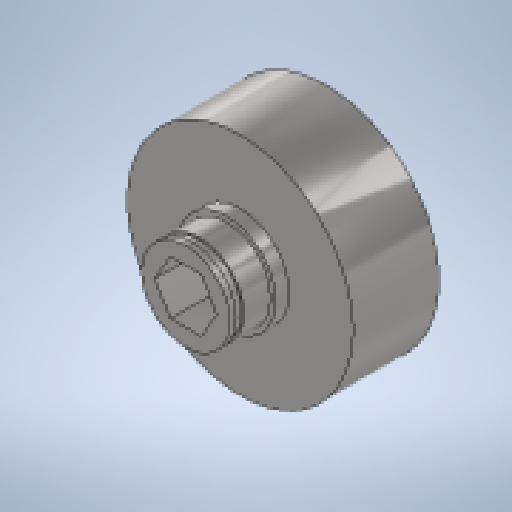
# Autodesk Inventor part: Clutch
Saved by Autodesk Inventor 2023.2 (Build 272271000, 271)
## iProperties
Created: 2024-03-17
Part Number: Clutch
Material: Stainless Steel
Document SubType Name: Modeling
Designer: Nathan Cai
Mass: 40.0707 g
Surface Area: 43.4565 cm^2
Volume: 5.00884 cm^3
Density: 8 g/cm^3
Appearance: Semi-Polished
Author: Nathan Cai
Autodesk Inventor part; units mm, degrees
ref_plane "YZ Plane" through (0, 0, 0) normal (1, 0, 0) x (0, 1, 0)
ref_plane "XZ Plane" through (0, 0, 0) normal (0, 1, 0) x (-1, 0, 0)
ref_plane "XY Plane" through (0, 0, 0) normal (0, 0, 1) x (1, 0, 0)
sketch "Sketch1" plane through (0, 0, 0) normal (1, 0, 0) x (0, 1, 0)
  line L0 (0, 0) -> (15.875, 0) construction
  line L1 (15.875, 0) -> (15.875, 9.525) construction
  line L2 (15.875, 9.525) -> (0, 9.525)
  line L3 (0, 9.525) -> (0, 0) construction
  line L4 (15.875, 0) -> (13.7634, 9.525)
  line L5 (0, 0) -> (16.6688, 0)
  line L6 (16.6688, 0) -> (16.6687, 12.7)
  line L7 (16.6687, 12.7) -> (0, 12.7)
  line L8 (0, 12.7) -> (0, 0)
  line L9 (0, 9.525) -> (6.5, 9.525)
  line L10 (6.5, 9.525) -> (6.5, 20.7266)
  line L11 (6.5, 20.7266) -> (0, 20.7266)
  line L12 (0, 20.7266) -> (0, 9.525)
  line L13 (0, 0) -> (3.9688, 0)
  line L14 (3.9688, 0) -> (3.9687, 20.7266)
  line L15 (3.9687, 20.7266) -> (0, 20.7266)
  line L16 (0, 20.7266) -> (0, 0)
  line L17 (6.5, 19.8) -> (6.2, 19.8)
  line L18 (6.2, 19.8) -> (6.2, 18.7)
  line L19 (6.2, 18.7) -> (6.5, 18.7)
  line L20 (6.5, 18.7) -> (6.5, 19.8)
  line L21 (6.5, 12.7) -> (7.25, 12.7)
  line L22 (7.25, 12.7) -> (7.25, 14.7)
  line L23 (7.25, 14.7) -> (6.5, 14.7)
  line L24 (6.5, 14.7) -> (6.5, 12.7)
  point P0 (3.9687, 9.525)
  dimension "d0" = 15.875
  dimension "d1" = 9.525
  dimension "d2" = 12.5
  dimension "d3" = 0.7937
  dimension "d4" = 12.7
  dimension "d5" = 6.5
  dimension "d6" = 3.9688
  dimension "d7" = 8.0266
  dimension "d8" = 0.3
  dimension "d9" = 1.1
  dimension "d10" = 6
  dimension "d12" = 0.75
  dimension "d13" = 2
  constraints: 50 end point, 12 parallel, 6 horizontal, 6 perpendicular, 5 point on line
  measures "d0" distance of L2.end L1.end
  measures "d1" distance of L1.end L0.end
  measures "d2" angle of L4 L1
  measures "d3" distance between parallel lines of L6 L1
  measures "d4" distance between parallel lines of L0 L7
  measures "d5" distance of L11.end L10.end
  measures "d6" distance between parallel lines of L16 L14
  measures "d7" distance between parallel lines of L7 L11
  measures "d8" distance of L19.end L18.end
  measures "d9" distance of L18.end L17.end
  measures "d10" distance between parallel lines of L7 L19
  measures "d12" distance of L23.end L22.end
  measures "d13" distance of L22.end L21.end
revolve "Revolution1" add sketch "Sketch1" angle 360 about axis through (0, 0, 12.7) along (0, 0, -1) contours L2 L10 L7 L6 L5 L4 | L2 L14 L7 L10 | L10 L23 L22 L7 | L7 L14 L11 L10 L17 L18 L19
sketch "Sketch2" plane through (0, 0, 20.7266) normal (0, 0, 1) x (1, 0, 0)
  circle A0 centre (0, 0) radius 3.9688 construction
  line L0 (2.2914, 3.9688) -> (4.5827, 0)
  line L1 (4.5827, 0) -> (2.2914, -3.9688)
  line L2 (2.2914, -3.9688) -> (-2.2914, -3.9687)
  line L3 (-2.2914, -3.9687) -> (-4.5827, 0)
  line L4 (-4.5827, 0) -> (-2.2914, 3.9688)
  line L5 (-2.2914, 3.9688) -> (2.2914, 3.9688)
  point P0 (0, 0)
  point P1 (0, 0)
  point P2 (0, 3.9687)
  constraints: 12 end point, 1 coincident, 1 horizontal, 1 midpoint, 1 vertical alignment, 14 other
extrude "Extrusion1" cut sketch "Sketch2" against normal through all
body "Solid1"
